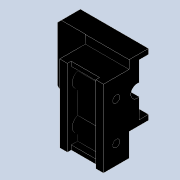
# Autodesk Inventor part: Y Axis Belt Adjustable and Plate Spacer
Saved by Autodesk Inventor 2022 (Build 260153000, 153)
## iProperties
Created: 2021-10-13
Part Number: Y Axis Belt Adjustable and Plate Spacer
Material: Generic
Document SubType Name: Modeling
Designer: Coy
Density: 1 g/cm^3
Appearance: Anodized - Black
Author: Coy
Autodesk Inventor part; units mm, degrees
ref_plane "YZ Plane" through (0, 0, 0) normal (1, 0, 0) x (0, 1, 0)
ref_plane "XZ Plane" through (0, 0, 0) normal (0, 1, 0) x (-1, 0, 0)
ref_plane "XY Plane" through (0, 0, 0) normal (0, 0, 1) x (1, 0, 0)
sketch "Sketch1" plane through (0, 0, 0) normal (1, 0, 0) x (0, 1, 0)
  line L0 (0, 0) -> (60, 0)
  line L1 (60, 0) -> (60, 20)
  line L2 (60, 20) -> (0, 20)
  line L3 (0, 20) -> (0, 0)
  line L4 (60, 10) -> (0, 10) construction
  line L5 (60, 10) -> (30, 10) construction
  line L6 (30, 10) -> (0, 10) construction
  circle A0 centre (45, 10) radius 2.75
  circle A1 centre (15, 10) radius 2.75
  dimension "d0" = 60
  dimension "d1" = 20
  dimension "d2" = 5.5
  dimension "d3" = 5.5
  constraints: 14 end point, 5 midpoint, 2 centre point, 2 parallel, 1 collinear, 1 horizontal, 1 perpendicular
  measures "d0" distance of L2.end L1.end
  measures "d1" distance of L1.end L0.end
  measures "d2" diameter of A0
  measures "d3" diameter of A1
extrude "Extrusion1" add sketch "Sketch1" against normal blind 6
sketch "Sketch2" plane through (-6, 0, 0) normal (-1, 0, 0) x (0, 0, 1)
  circle A0 centre (10, 45) radius 2.75 projected
  circle A1 centre (10, 15) radius 2.75 projected
  circle A2 centre (10, 45) radius 6.25
  circle A3 centre (10, 15) radius 6.25
  line L0 (20, 60) -> (0, 60) projected
  line L1 (12, 60) -> (12, 0)
  line L2 (8, 60) -> (8, 0)
  line L3 (0, 0) -> (20, 0) projected
  line L4 (0, 60) -> (0, 0) projected
  line L5 (20, 0) -> (20, 60) projected
  line L6 (12, 56.5) -> (17, 56.5)
  line L7 (17, 56.5) -> (17, 60)
  line L8 (8, 56.5) -> (3, 56.5)
  line L9 (3, 56.5) -> (3, 60)
  line L10 (8, 3.5) -> (3, 3.5)
  line L11 (3, 3.5) -> (3, 0)
  line L12 (12, 3.5) -> (17, 3.5)
  line L13 (17, 3.5) -> (17, 0)
  point P0 (12, 39.0786)
  point P1 (12, 50.9214)
  point P2 (8, 50.9214)
  point P3 (8, 39.0786)
  point P4 (8, 20.9214)
  point P5 (8, 9.0786)
  point P6 (12, 9.0786)
  point P7 (12, 20.9214)
  dimension "d6" = 3.5
  dimension "d7" = 8
  dimension "d8" = 8
  dimension "d9" = 3.5
  dimension "d10" = 3.5
  dimension "d11" = 3.5
  dimension "d16" = 3.5
  constraints: 20 end point, 15 point on line, 4 perpendicular, 2 centre point, 2 horizontal, 2 vertical, 1 coincident
  measures "d6" radial gap between concentric circles of A0 A2
  measures "d7" distance between parallel lines of L4 L2
  measures "d8" distance between parallel lines of L5 L1
  measures "d9" distance of L6.end L7.end
  measures "d10" distance of L8.end L9.end
  measures "d11" distance of L12.end L13.end
  measures "d16" radial gap between concentric circles of A1 A3
extrude "Extrusion2" add sketch "Sketch2" along normal blind 22.1 contours A0 L1 A2 | A0 L2 A2 L1 | L1 A2 L2 A0 | A0 L2 A2 | A2 L2 L0 L1 | L1 A3 L2 A2 | A2 L2 A3 L10 L11 L3 L4 L0 L9 L8 | L1 L0 L7 L6 | L1 A1 L2 A3 | A3 L1 A1 | L8 L9 L0 L2 | L2 A1 A3 | L2 A1 L1 A3 | A3 L1 L3 L2 | L2 L3 L11 L10 | L12 L13 L3 L1
sketch "Sketch3" plane through (-28.1, 0, 0) normal (-1, 0, 0) x (0, 0, 1)
  circle A0 centre (10, 45) radius 2.75 projected
  circle A1 centre (10, 15) radius 2.75 projected
  line L0 (20, 0) -> (20, 60) projected
  line L1 (0, 0) -> (20, 0) projected
  line L2 (0, 0) -> (20, 0) projected
  line L3 (0, 0) -> (20, 0) projected
  line L4 (0, 60) -> (0, 0) projected
  line L5 (20, 60) -> (17, 60) projected
  line L6 (20, 60) -> (0, 60) projected
  line L7 (20, 60) -> (17, 60) projected
  point P0 (17, 0)
  point P1 (3, 0)
  point P2 (3, 60)
extrude "Extrusion3" add sketch "Sketch3" along normal blind 6
sketch "Sketch4" plane through (0, 0, 0) normal (0, 0, -1) x (-1, 0, 0)
  line L0 (0, 60) -> (0, 0) projected
  line L1 (34.1, 60) -> (34.1, 0) projected
  line L2 (0, 60) -> (34.1, 60)
  line L3 (34.1, 60) -> (34.1, 24.6)
  line L4 (34.1, 24.6) -> (0, 24.6)
  line L5 (0, 24.6) -> (0, 60)
  line L6 (34.1, 0) -> (34.1, 60) projected
  line L7 (0, 0) -> (0, 60) projected
  line L8 (34.1, 62.55) -> (0, 62.55)
  line L9 (0, 62.55) -> (0, 22.05)
  line L10 (0, 22.05) -> (34.1, 22.05)
  line L11 (34.1, 22.05) -> (34.1, 62.55)
  line L12 (0, 66.55) -> (34.1, 66.55)
  line L13 (34.1, 18.05) -> (0, 18.05)
  line L14 (2.6912, 62.55) -> (2.6912, 22.05) construction
  line L15 (34.1, 62.55) -> (34.1, 66.55)
  line L16 (0, 62.55) -> (0, 66.55)
  point P0 (34.1, 54.55)
  point P1 (0, 54.55)
  point P2 (2.6912, 42.3)
  dimension "d17" = 35.4
  dimension "d18" = 40.5
  dimension "d20" = 4
  dimension "d45" = 17.7
  dimension "d46" = 4
  constraints: 26 end point, 9 point on line, 5 parallel, 3 perpendicular, 2 horizontal, 2 vertical, 1 midpoint
  measures "d17" distance of L2.end L3.end
  measures "d18" distance of L9.end L8.end
  measures "d20" distance between parallel lines of L8 L12
  measures "d45" distance from line of L2 point (2.691, 42.3)
  measures "d46" distance between parallel lines of L10 L13
extrude "Extrusion4" add sketch "Sketch4" along normal blind 7.847
sketch "Sketch5" plane through (0, 0, -7.847) normal (0, 0, -1) x (-1, 0, 0)
  line L0 (34.1, 18.05) -> (34.1, 66.55) projected
  line L1 (34.1, 66.55) -> (0, 66.55) projected
  line L2 (0, 66.55) -> (0, 18.05) projected
  line L3 (0, 18.05) -> (34.1, 18.05) projected
  line L4 (34.1, 18.05) -> (34.1, 54.55) projected
  line L5 (0, 54.55) -> (0, 18.05) projected
  line L6 (34.1, 62.55) -> (0, 62.55)
  line L7 (0, 62.55) -> (0, 22.05)
  line L8 (0, 22.05) -> (34.1, 22.05)
  line L9 (34.1, 22.05) -> (34.1, 62.55)
  point P0 (0, 0)
  point P1 (0, 62.55)
  point P2 (34.1, 22.05)
  dimension "d23" = 40.5
  dimension "d24" = 4
  constraints: 8 end point, 2 parallel, 2 point on line, 1 horizontal, 1 perpendicular
  measures "d23" distance of L7.end L6.end
  measures "d24" distance between parallel lines of L3 L8
extrude "Extrusion5" add sketch "Sketch5" along normal blind 7.28 contours L3 L2 L8 L0 | L6 L2 L1 L0
sketch "Sketch6" plane through (0, 0, 0) normal (1, 0, 0) x (0, 0, -1)
  line L0 (7.847, 22.05) -> (15.127, 22.05) construction
  line L1 (7.847, 62.55) -> (15.127, 62.55) construction
  line L2 (7.847, 22.05) -> (10.847, 22.05) construction
  line L3 (10.847, 22.05) -> (10.847, 62.55) construction
  line L4 (10.847, 62.55) -> (7.847, 62.55) construction
  line L5 (7.847, 62.55) -> (7.847, 22.05) construction
  line L6 (7.847, 22.05) -> (7.847, 62.55) construction
  line L7 (7.847, 42.3) -> (1.4795, 42.3) construction
  circle A0 centre (6.347, 42.3) radius 2.5 construction
  circle A1 centre (6.347, 42.3) radius 4.5
  line L8 (0, 60) -> (-20, 60) projected
  line L9 (-20, 60) -> (-20, 0) projected
  line L10 (-20, 0) -> (0, 0) projected
  line L11 (0, 0) -> (0, 18.05) projected
  circle A2 centre (-10, 45) radius 2.75 projected
  circle A3 centre (-10, 15) radius 2.75 projected
  circle A4 centre (6.347, 42.3) radius 5
  line L12 (0, 18.05) -> (15.127, 18.05) projected
  line L13 (15.127, 22.05) -> (15.127, 18.05) projected
  line L14 (7.847, 22.05) -> (15.127, 22.05) projected
  line L15 (7.847, 62.55) -> (7.847, 22.05) projected
  line L16 (7.847, 62.55) -> (15.127, 62.55) projected
  line L17 (15.127, 66.55) -> (15.127, 62.55) projected
  line L18 (0, 66.55) -> (15.127, 66.55) projected
  line L19 (0, 66.55) -> (0, 60) projected
  point P0 (7.847, 47.0697)
  point P1 (7.847, 37.5303)
  dimension "d27" = 3
  dimension "d28" = 5
  dimension "d29" = 2
  dimension "d30" = 2
  dimension "d31" = 0.5
  constraints: 10 end point, 3 centre point, 2 horizontal, 2 parallel, 2 point on line, 1 midpoint, 1 perpendicular
  measures "d27" distance of L4.end L3.end
  measures "d28" diameter of A0
  measures "d29" distance edge to line of A0 L3
  measures "d30" radial gap between concentric circles of A0 A1
  measures "d31" radial gap between concentric circles of A1 A4
extrude "Extrusion6" cut sketch "Sketch6" against normal through all contours L15 A1 | A1 L15 A4 picked at (4.8498, 43.4746) picked at (1.5593, 41.9128)
sketch "Sketch8" plane through (-34.1, 0, 0) normal (-1, 0, 0) x (0, 0, 1)
  line L0 (0, 18.05) -> (0, 0) projected
  line L1 (0, 0) -> (20, 0) projected
  line L2 (20, 0) -> (20, 60) projected
  line L3 (20, 60) -> (0, 60) projected
  circle A0 centre (10, 45) radius 2.75 projected
  circle A1 centre (10, 15) radius 2.75 projected
  line L4 (-0.2, 66.55) -> (-0.2, 18.05)
  line L5 (0, 18.05) -> (-15.127, 18.05) projected
  line L6 (0, 60) -> (0, 66.55) projected
  line L7 (0, 66.55) -> (-15.127, 66.55) projected
  line L8 (-15.127, 62.55) -> (-15.127, 66.55) projected
  line L9 (-7.847, 62.55) -> (-15.127, 62.55) projected
  line L10 (-7.847, 22.05) -> (-7.847, 37.5303) projected
  line L11 (-7.847, 22.05) -> (-15.127, 22.05) projected
  line L12 (-15.127, 18.05) -> (-15.127, 22.05) projected
  line L13 (0, 18.05) -> (-15.127, 18.05) projected
  arc A2 (-7.847, 37.5303) -> (-7.847, 47.0697) centre (-6.347, 42.3) ccw projected
  arc A3 (-7.847, 37.5303) -> (-7.847, 47.0697) centre (-6.347, 42.3) ccw projected
  line L14 (-7.847, 47.0697) -> (-7.847, 62.55) projected
  dimension "d34" = 0.2
  constraints: 2 end point, 2 point on line
  measures "d34" distance between parallel lines of L0 L4
extrude "Extrusion7" add sketch "Sketch8" along normal blind 17 contours L5 L12 L11 L10 A2 L14 L9 L8 L7 L4
sketch "Sketch9" plane through (-51.1, 0, 0) normal (-1, 0, 0) x (0, 0, 1)
  line L0 (-15.127, 22.05) -> (-15.127, 18.05) projected
  line L1 (-0.2, 18.05) -> (-0.2, 66.55) projected
  line L2 (-15.127, 22.05) -> (-15.127, 18.05) projected
  line L3 (-15.127, 18.05) -> (-15.127, 62.55)
  line L4 (-15.127, 62.55) -> (-7.847, 62.55) projected
  line L5 (-7.847, 37.5303) -> (-7.847, 22.05) projected
  line L6 (-7.847, 22.05) -> (-15.127, 22.05) projected
  line L7 (-15.127, 18.05) -> (-0.2, 18.05) projected
  line L8 (-0.2, 66.55) -> (-15.127, 66.55) projected
  line L9 (-15.127, 66.55) -> (-15.127, 62.55) projected
  arc A0 (-7.847, 37.5303) -> (-7.847, 47.0697) centre (-6.347, 42.3) ccw projected
  line L10 (-7.847, 62.55) -> (-7.847, 47.0697) projected
  point P0 (0, 0)
  point P1 (-15.127, 22.05)
  constraints: 2 end point, 1 collinear, 1 point on line
extrude "Extrusion8" add sketch "Sketch9" along normal blind 5
sketch "Sketch10" plane through (-56.1, 0, 0) normal (-1, 0, 0) x (0, 0, 1)
  arc A0 (-7.847, 37.5303) -> (-7.847, 47.0697) centre (-6.347, 42.3) ccw projected
  circle A1 centre (-6.347, 42.3) radius 2.6
  point P0 (0, 0)
  dimension "d39" = 5.2
  constraints: 1 centre point, 1 coincident
  measures "d39" diameter of A1
extrude "Extrusion9" cut sketch "Sketch10" against normal up to next
chamfer "Chamfer1" distance 3 angle 45 2 edges at (-56.1, 66.55, -7.6635) (-56.1, 18.05, -7.6635)
equation "\"d3\" = d2"
equation "\"d16\" = d6"
equation "\"d46\" = d20"
body "Solid1"
